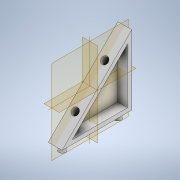
# Autodesk Inventor part: Roof_Wall_Small
Saved by Autodesk Inventor 2022.4 (Build 264492010, 492A)
## iProperties
Created: 2025-02-20
Part Number: Roof_Wall_Small
Material: Generic
Document SubType Name: Modeling
Designer: jan-m
Density: 1 g/cm^3
Appearance: Default
Author: jan-m
Autodesk Inventor part; units mm, degrees
sketch "Sketch2" plane through (0, 0, 0) normal (1, 0, 0) x (0, 1, 0)
  line L0 (25, 25) -> (-25, 25)
  line L1 (-25, 25) -> (-25, -25)
  line L2 (-25, -25) -> (25, -25)
  line L3 (25, -25) -> (25, 25)
  line L4 (-35, 0) -> (35, 0) projected
  line L5 (0, 35) -> (0, -35) projected
  line L6 (-25, 25) -> (25, -25)
  point P0 (0, 0)
  point P1 (25, 0)
  point P2 (0, 25)
  dimension "d0" = 50
  dimension "d1" = 50
  constraints: 10 end point, 2 midpoint, 2 parallel, 2 point on line, 1 horizontal, 1 perpendicular
  measures "d0" distance of L2.end L0.start
  measures "d1" distance of L1.end L2.end
extrude "Extrusion1" add sketch "Sketch2" along normal mid plane 10 contours L6 L4 L1 | L5 L2 L1 L4 | L6 L2 L5
sketch "Sketch4" plane through (5, 0, 0) normal (1, 0, 0) x (0, 0, -1)
  line L0 (25, 25) -> (-25, -25) projected
  line L1 (25, -25) -> (25, 25) projected
  line L2 (-25, -25) -> (25, -25) projected
  line L3 (22, 17.7574) -> (-17.7574, -22)
  line L4 (-17.7574, -22) -> (22, -22)
  line L5 (22, -22) -> (22, 17.7574)
  point P0 (0, 0)
  dimension "d8" = 3
  constraints: 6 end point, 2 other
  measures "d8" distance between parallel lines of L1 L5
extrude "Extrusion2" cut sketch "Sketch4" against normal blind 7 contours L5 L4 L3
sketch "Sketch5" plane through (-5, -25, -25) normal (0, -1, 0) x (1, 0, 0)
  line L0 (5, 60) -> (5, -10) projected
  circle A0 centre (5, 45) radius 2.5
  line L1 (10, 50) -> (0, 50) projected
  circle A1 centre (5, 5) radius 2.5
  point P0 (5, 25)
  dimension "d11" = 5
  dimension "d12" = 5
  dimension "d15" = 40
  constraints: 2 centre point, 1 point on line, 1 vertical, 2 other
  measures "d11" diameter of A0
  measures "d12" distance from line of L1 A0.centre
  measures "d15" distance of A0.centre A1.centre
extrude "Extrusion3" add sketch "Sketch5" along normal blind 5
sketch "Sketch8" plane through (-5, -25, 25) normal (0, 0.7071068, 0.7071068) x (1, 0, 0)
  line L0 (10, 0) -> (0, 0) projected
  line L1 (0, 70.7107) -> (10, 70.7107) projected
  circle A0 centre (5, 50.3553) radius 2.5
  line L2 (5, 84.8528) -> (5, -14.1421) projected
  line L3 (-2, 35.3553) -> (12, 35.3553) projected
  circle A1 centre (5, 20.3553) radius 2.5
  point P0 (5, 35.3553)
  dimension "d31" = 70.7107
  dimension "d32" = 5
  dimension "d34" = 15
  constraints: 2 centre point, 1 point on line, 1 symmetric about line, 1 other
  measures "d31" distance between parallel lines of L0 L1
  measures "d32" diameter of A0
  measures "d34" distance from line of L3 A0.centre
extrude "Extrusion4" cut sketch "Sketch8" against normal blind 7
body "Solid1"
